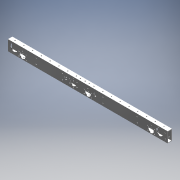
# Autodesk Inventor part: Main Extrusion
Saved by Autodesk Inventor 2019.4 (Build 234330000, 330)
## iProperties
Created: 2020-01-05
Part Number: Main Extrusion
Material: Aluminum 6061
Document SubType Name: Modeling
Designer: Mark
Mass: 1095.18 g
Surface Area: 2784.42 cm^2
Volume: 405.623 cm^3
Density: 2.7 g/cm^3
Appearance: Aluminum - Flat
Author: Mark
Autodesk Inventor part; units mm, degrees
ref_plane "YZ Plane" through (0, 0, 0) normal (1, 0, 0) x (0, 1, 0)
ref_plane "XZ Plane" through (0, 0, 0) normal (0, 1, 0) x (-1, 0, 0)
ref_plane "XY Plane" through (0, 0, 0) normal (0, 0, 1) x (1, 0, 0)
sketch "Sketch1" plane through (0, 0, 0) normal (1, 0, 0) x (0, 1, 0)
  line L0 (-30, 12.5) -> (30, 12.5)
  line L1 (30, 12.5) -> (30, -12.5)
  line L2 (30, -12.5) -> (-30, -12.5)
  line L3 (-30, -12.5) -> (-30, 12.5)
  line L4 (-30, 12.5) -> (30, -12.5) construction
  line L5 (30, 12.5) -> (-30, -12.5) construction
  line L6 (-27, 9.5) -> (27, 9.5)
  line L7 (27, 9.5) -> (27, -9.5)
  line L8 (27, -9.5) -> (-27, -9.5)
  line L9 (-27, -9.5) -> (-27, 9.5)
  line L10 (-27, 9.5) -> (27, -9.5) construction
  line L11 (27, 9.5) -> (-27, -9.5) construction
  point P0 (0, 0)
  dimension "d0" = 60
  dimension "d1" = 25
  dimension "d2" = 54
  dimension "d3" = 19
  constraints: 24 end point, 4 midpoint, 4 parallel, 2 horizontal, 2 perpendicular
  measures "d0" distance of L1.end L2.end
  measures "d1" distance of L0.end L1.end
  measures "d2" distance of L7.end L8.end
  measures "d3" distance of L6.end L7.end
extrude "Extrusion1" add sketch "Sketch1" along normal blind 910
sketch "Sketch2" plane through (0, -30, 12.5) normal (0, 0, 1) x (1, 0, 0)
  circle A0 centre (455, 20) radius 16
  circle A1 centre (82.3802, 20) radius 16
  circle A2 centre (815, 20) radius 16
  line L0 (0, 0) -> (0, 60) projected
  line L1 (0, 0) -> (910, 0) projected
  circle A3 centre (372.2077, 30) radius 16
  circle A4 centre (455, 20) radius 23.5 construction
  line L2 (455, 20) -> (455, -3.5) construction
  line L3 (455, 20) -> (478.5, 20) construction
  circle A5 centre (455, -3.5) radius 2.75
  circle A6 centre (475.3516, 8.25) radius 2.75
  circle A7 centre (475.3516, 31.75) radius 2.75
  circle A8 centre (455, 43.5) radius 2.75
  circle A9 centre (434.6484, 31.75) radius 2.75
  circle A10 centre (434.6484, 8.25) radius 2.75
  circle A11 centre (372.2077, 30) radius 23.5 construction
  line L4 (372.2077, 30) -> (372.2077, 6.5) construction
  line L5 (372.2077, 30) -> (395.7077, 30) construction
  circle A12 centre (392.5593, 18.25) radius 2.75
  circle A13 centre (392.5593, 41.75) radius 2.75
  circle A14 centre (372.2077, 53.5) radius 2.75
  circle A15 centre (351.8561, 41.75) radius 2.75
  circle A16 centre (351.8561, 18.25) radius 2.75
  circle A17 centre (372.2077, 6.5) radius 2.75
  circle A18 centre (82.3802, 20) radius 23.5 construction
  line L6 (82.3802, 20) -> (82.3802, -3.5) construction
  line L7 (82.3802, 20) -> (105.8802, 20) construction
  circle A19 centre (82.3802, -3.5) radius 2.75
  circle A20 centre (102.7318, 8.25) radius 2.75
  circle A21 centre (102.7318, 31.75) radius 2.75
  circle A22 centre (82.3802, 43.5) radius 2.75
  circle A23 centre (62.0286, 31.75) radius 2.75
  circle A24 centre (62.0286, 8.25) radius 2.75
  circle A25 centre (815, 20) radius 23.5 construction
  line L8 (815, 20) -> (815, -3.5) construction
  circle A26 centre (815, -3.5) radius 2.75
  circle A27 centre (835.3516, 8.25) radius 2.75
  circle A28 centre (835.3516, 31.75) radius 2.75
  circle A29 centre (815, 43.5) radius 2.75
  circle A30 centre (794.6484, 31.75) radius 2.75
  circle A31 centre (794.6484, 8.25) radius 2.75
  circle A32 centre (331.1877, 34) radius 4.25
  circle A33 centre (497.2277, 34) radius 4.25
  point P0 (0, 30)
  dimension "d22" = 47
  dimension "d36" = 47
  dimension "d43" = 47
  dimension "d6" = 32
  dimension "d7" = 32
  dimension "d8" = 32
  dimension "d9" = 455
  dimension "d10" = 20
  dimension "d13" = 20
  dimension "d14" = 20
  dimension "d18" = 32
  dimension "d19" = 30
  dimension "d20" = 83.394
  dimension "d21" = 290
  dimension "d23" = 90
  dimension "d24" = 5.5
  dimension "d27" = 360
  dimension "d29" = 47
  dimension "d30" = 90
  dimension "d31" = 5.5
  dimension "d34" = 360
  dimension "d37" = 90
  dimension "d38" = 5.5
  dimension "d41" = 360
  dimension "d44" = 360
  dimension "d45" = 5.5
  dimension "d48" = 360
  dimension "d82" = 8.5
  dimension "d83" = 41.02
  dimension "d84" = 4
  dimension "d85" = 8.5
  dimension "d87" = 4
  dimension "d96" = 166.04
  constraints: 31 centre point, 14 end point, 8 coincident, 3 horizontal, 3 perpendicular, 3 vertical alignment, 2 point on circle, 1 vertical, 58 other
  measures "d6" diameter of A0
  measures "d7" diameter of A1
  measures "d8" diameter of A2
  measures "d9" distance from line of L0 A0.centre
  measures "d10" distance from line of L1 A0.centre
  measures "d13" distance from line of L1 A1.centre
  measures "d14" distance from line of L1 A2.centre
  measures "d18" diameter of A3
  measures "d19" distance from line of L1 A3.centre
  measures "d20" distance of A0.centre A3.centre
  measures "d21" distance of A3.centre A1.centre
  measures "d23" angle of L2 L3
  measures "d24" diameter of A5
  measures "d29" diameter of A11
  measures "d30" angle of L4 L5
  measures "d31" diameter of A12
  measures "d37" angle of L6 L7
  measures "d38" diameter of A19
  measures "d44" distance of A0.centre A2.centre
  measures "d45" diameter of A26
  measures "d82" diameter of A32
  measures "d83" horizontal distance of A3.centre A32.centre
  measures "d84" vertical distance of A32.centre A3.centre
  measures "d85" diameter of A33
  measures "d87" vertical distance of A3.centre A33.centre
  measures "d96" distance of A33.centre A32.centre
extrude "Extrusion2" cut sketch "Sketch2" against normal blind 30 contours A0 | A1 | A2 | A3 | A6 | A7 | A8 | A9 | A10 | A12 | A13 | A14 | A15 | A16 | A17 | A20 | A21 | A22 | A23 | A24 | A27 | A28 | A29 | A30 | A31 | A32 | A33
sketch "Sketch3" plane through (0, -30, -12.5) normal (0, -1, 0) x (1, 0, 0)
  circle A0 centre (27.5, 12.5) radius 2.75
  line L0 (0, 25) -> (910, 25) projected
  line L1 (0, 0) -> (0, 25) projected
  circle A1 centre (77.5, 12.5) radius 2.75
  circle A2 centre (127.5, 12.5) radius 2.75
  circle A3 centre (177.5, 12.5) radius 2.75
  circle A4 centre (227.5, 12.5) radius 2.75
  circle A5 centre (277.5, 12.5) radius 2.75
  circle A6 centre (327.5, 12.5) radius 2.75
  circle A7 centre (377.5, 12.5) radius 2.75
  circle A8 centre (427.5, 12.5) radius 2.75
  circle A9 centre (477.5, 12.5) radius 2.75
  circle A10 centre (527.5, 12.5) radius 2.75
  circle A11 centre (577.5, 12.5) radius 2.75
  circle A12 centre (627.5, 12.5) radius 2.75
  circle A13 centre (677.5, 12.5) radius 2.75
  circle A14 centre (727.5, 12.5) radius 2.75
  circle A15 centre (777.5, 12.5) radius 2.75
  circle A16 centre (827.5, 12.5) radius 2.75
  circle A17 centre (877.5, 12.5) radius 2.75
  circle A18 centre (927.5, 12.5) radius 2.75
  circle A19 centre (977.5, 12.5) radius 2.75
  point P0 (0, 12.5)
  dimension "d50" = 5.5
  dimension "d51" = 12.5
  dimension "d52" = 27.5
  dimension "d55" = 50
  constraints: 20 centre point, 1 horizontal, 38 other
  measures "d50" diameter of A0
  measures "d51" distance from line of L0 A0.centre
  measures "d52" distance from line of L1 A0.centre
  measures "d55" distance of A0.centre A1.centre
extrude "Extrusion3" cut sketch "Sketch3" against normal blind 60 contours A0 | A1 | A2 | A3 | A4 | A5 | A6 | A7 | A8 | A9 | A10 | A11 | A12 | A13 | A14 | A15 | A16 | A17
sketch "Sketch4" plane through (0, -30, 12.5) normal (0, 0, 1) x (1, 0, 0)
  circle A0 centre (160, 45) radius 2.75
  line L0 (0, 60) -> (910, 60) projected
  line L1 (0, 0) -> (0, 60) projected
  circle A1 centre (160, 15) radius 2.75
  line L2 (0, 0) -> (910, 0) projected
  circle A2 centre (735, 45) radius 2.75
  circle A3 centre (735, 15) radius 2.75
  circle A4 centre (895, 45) radius 2.75
  circle A5 centre (895, 15) radius 2.75
  line L3 (910, 60) -> (910, 0) projected
  circle A6 centre (310, 45) radius 2.75
  circle A7 centre (310, 15) radius 2.75
  circle A8 centre (540, 45) radius 2.75
  circle A9 centre (540, 15) radius 2.75
  point P0 (0, 30)
  dimension "d62" = 5.5
  dimension "d63" = 15
  dimension "d64" = 160
  dimension "d65" = 5.5
  dimension "d66" = 15
  dimension "d67" = 160
  dimension "d68" = 5.5
  dimension "d69" = 5.5
  dimension "d70" = 5.5
  dimension "d71" = 5.5
  dimension "d72" = 15
  dimension "d73" = 15
  dimension "d74" = 15
  dimension "d75" = 15
  dimension "d76" = 15
  dimension "d77" = 15
  dimension "d78" = 160
  dimension "d79" = 160
  dimension "d97" = 5.5
  dimension "d98" = 5.5
  dimension "d99" = 5.5
  dimension "d100" = 5.5
  dimension "d101" = 15
  dimension "d102" = 15
  dimension "d103" = 15
  dimension "d104" = 15
  dimension "d105" = 310
  dimension "d106" = 310
  dimension "d107" = 370
  dimension "d108" = 370
  constraints: 10 centre point
  measures "d62" diameter of A0
  measures "d63" distance from line of L0 A0.centre
  measures "d64" distance from line of L1 A0.centre
  measures "d65" diameter of A1
  measures "d66" distance from line of L2 A1.centre
  measures "d67" distance from line of L1 A1.centre
  measures "d68" diameter of A2
  measures "d69" diameter of A3
  measures "d70" diameter of A4
  measures "d71" diameter of A5
  measures "d72" distance from line of L0 A4.centre
  measures "d73" distance from line of L0 A2.centre
  measures "d74" distance from line of L2 A3.centre
  measures "d75" distance from line of L2 A5.centre
  measures "d76" distance from line of L3 A4.centre
  measures "d77" distance from line of L3 A5.centre
  measures "d78" distance of A4.centre A2.centre
  measures "d79" distance of A5.centre A3.centre
  measures "d97" diameter of A6
  measures "d98" diameter of A7
  measures "d99" diameter of A8
  measures "d100" diameter of A9
  measures "d101" distance from line of L2 A9.centre
  measures "d102" distance from line of L0 A8.centre
  measures "d103" distance from line of L0 A6.centre
  measures "d104" distance from line of L2 A7.centre
  measures "d105" distance from line of L1 A7.centre
  measures "d106" distance from line of L1 A6.centre
  measures "d107" distance from line of L3 A8.centre
  measures "d108" distance from line of L3 A9.centre
extrude "Extrusion4" cut sketch "Sketch4" against normal blind 60 contours A0 | A1 | A2 | A3 | A4 | A5 | A6 | A7 | A8 | A9
sketch "Sketch5" plane through (0, -30, -12.5) normal (0, -1, 0) x (1, 0, 0)
  circle A0 centre (400.333, 12.5) radius 2.75
  circle A1 centre (377.5, 12.5) radius 2.75 projected
  line L0 (0, 0) -> (910, 0) projected
  circle A2 centre (450.333, 12.5) radius 2.75
  point P0 (0, 12.5)
  dimension "d88" = 5.5
  dimension "d89" = 22.833
  dimension "d90" = 12.5
  dimension "d91" = 5.5
  dimension "d92" = 50
  dimension "d93" = 12.5
  constraints: 2 centre point
  measures "d88" diameter of A0
  measures "d89" distance of A1.centre A0.centre
  measures "d90" distance from line of L0 A0.centre
  measures "d91" diameter of A2
  measures "d92" distance of A0.centre A2.centre
  measures "d93" distance from line of L0 A2.centre
extrude "Extrusion5" cut sketch "Sketch5" against normal blind 60 contours A0 | A2
sketch "Sketch6" plane through (0, -30, 12.5) normal (0, 0, 1) x (1, 0, 0)
  circle A0 centre (497.2277, 34) radius 4.25 projected
  circle A1 centre (331.1877, 34) radius 4.25 projected
  point P0 (0, 30)
  constraints: 2 coincident
hole "Hole1" at (497.2277, 4, 12.5) at (331.1877, 4, 12.5) direction (0, 0, -1) diameter 18 depth 8
sketch "Sketch7" plane through (0, -30, 12.5) normal (0, 0, 1) x (1, 0, 0)
  circle A0 centre (35, 35) radius 20
  line L0 (0, 0) -> (910, 0) projected
  line L1 (0, 0) -> (0, 60) projected
  circle A1 centre (865, 35) radius 20
  line L2 (910, 60) -> (910, 0) projected
  point P0 (0, 30)
  dimension "d116" = 40
  dimension "d117" = 35
  dimension "d118" = 35
  dimension "d119" = 40
  dimension "d120" = 45
  dimension "d121" = 35
  constraints: 2 centre point
  measures "d116" diameter of A0
  measures "d117" distance from line of L0 A0.centre
  measures "d118" distance from line of L1 A0.centre
  measures "d119" diameter of A1
  measures "d120" distance from line of L2 A1.centre
  measures "d121" distance from line of L0 A1.centre
extrude "Extrusion6" cut sketch "Sketch7" against normal blind 10
equation "\"d13\" = d10"
equation "\"d14\" = d10"
equation "\"d66\" = d63"
equation "\"d67\" = d64"
equation "\"d72\" = d63"
equation "\"d73\" = d63"
equation "\"d74\" = d63"
equation "\"d75\" = d63"
equation "\"d77\" = d76"
equation "\"d79\" = d78"
equation "\"d101\" = d63"
equation "\"d102\" = d63"
equation "\"d103\" = d63"
equation "\"d104\" = d63"
body "Solid1"
